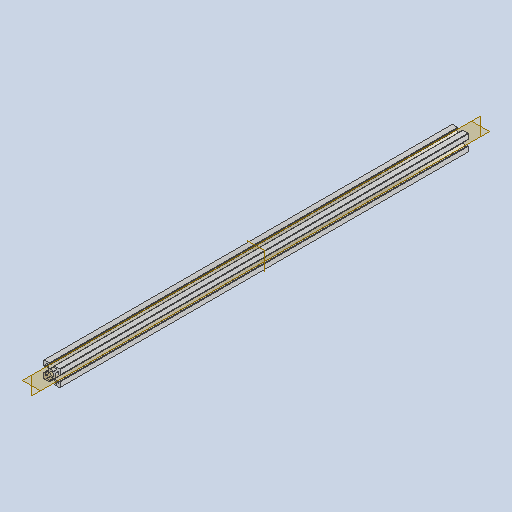
# Autodesk Inventor part: PERFIL_20X20_001
Saved by Autodesk Inventor 2026 (Build 300175000, 175)
## iProperties
Created: 2025-03-25
Part Number: PERFIL_20X20_001
Material: Alumínio 6061
Document SubType Name: Modeling
Designer: Carlos Dias
Density: 2.7 g/cm^3
Appearance: Alumínio - Polido
Description: 50x20
Author: Carlos Dias
Autodesk Inventor part; units mm, degrees
sketch "Esboço1" plane through (0, 0, 0) normal (0, 0, 1) x (1, 0, 0)
  line L0 (-10, 10) -> (10, 10) construction
  circle A0 centre (0, 0) radius 2.5
  line L1 (-4, 4) -> (4, 4) construction
  line L2 (-10, 10) -> (0, 0) construction
  line L3 (-4, 4) -> (-4, -4) construction
  line L4 (-6.5858, 8) -> (-2.5858, 4) construction
  line L5 (-6.5858, 8) -> (-2.5858, 8) construction
  line L6 (-2.5858, 8) -> (-2.5858, 10) construction
  line L7 (-2.5858, 10) -> (-3.0858, 10) construction
  line L8 (-3.0858, 10) -> (-3.0858, 9.5)
  line L9 (-3.0858, 9.5) -> (-2.5858, 9.5)
  line L10 (-2.5858, 9.5) -> (-2.5858, 10) construction
  line L11 (-8, 6.5858) -> (-4, 2.5858) construction
  line L12 (-2.5858, 8) -> (-2.5858, 9.5)
  line L13 (-3.0858, 10) -> (-10, 10)
  line L14 (-10, 10) -> (-10, 3.0858) construction
  line L15 (-10, 3.0858) -> (-8, 3.0858) construction
  line L16 (-8, 6.5858) -> (-8, 3.0858) construction
  line L17 (-10, 3.0858) -> (-9.5, 3.0858) construction
  line L18 (-9.5, 3.0858) -> (-9.5, 3.5858)
  line L19 (-9.5, 3.5858) -> (-10, 3.5858)
  line L20 (-10, 3.5858) -> (-10, 3.0858) construction
  line L21 (-8, 3.0858) -> (-9.5, 3.0858)
  arc A1 (-2.7322, 4.1464) -> (-2.3787, 4) centre (-2.3787, 4.5) ccw
  line L22 (-2.3787, 4) -> (0, 4)
  arc A2 (-5.8615, 8) -> (-6.0737, 7.4879) centre (-5.8615, 7.7) ccw
  line L23 (-6.0737, 7.4879) -> (-2.7322, 4.1464)
  line L24 (-5.8615, 8) -> (-2.5858, 8)
  arc A3 (-4, 2.3787) -> (-4.1464, 2.7322) centre (-4.5, 2.3787) ccw
  arc A4 (-7.4879, 6.0737) -> (-8, 5.8615) centre (-7.7, 5.8615) ccw
  line L25 (-8, 5.8615) -> (-8, 3.0858)
  line L26 (-7.4879, 6.0737) -> (-4.1464, 2.7322)
  arc A5 (-9.5, 10) -> (-10, 9.5) centre (-9.5, 9.5) ccw
  line L27 (-4, 2.3787) -> (-4, 0)
  line L28 (-10, 9.5) -> (-10, 3.5858)
  line L29 (-4, 0) -> (0, 0)
  line L30 (0, 4) -> (0, 0)
  point P0 (0, 10)
  point P1 (-5, 5)
  point P2 (-10, 6.5429)
  point P3 (-2.5, 0)
  point P4 (0, 2.5)
  dimension "d1" = 20
  dimension "d2" = 10
  dimension "d3" = 5
  dimension "d4" = 6
  dimension "d5" = 1
  dimension "d7" = 2
  dimension "d8" = 0.5
  dimension "d9" = 1
  dimension "d10" = 2
  dimension "d12" = 0.5
  dimension "d13" = 0.3
  dimension "d14" = 0.5
  dimension "d15" = 0.3
  dimension "d16" = 0.5
  dimension "d17" = 8
  constraints: 62 end point, 14 point on line, 10 point on circle, 10 tangent, 8 perpendicular, 7 horizontal, 6 centre point, 6 collinear, 6 parallel, 5 midpoint, 4 vertical, 3 coincident, 3 vertical alignment
  measures "d1" distance of L0.start L0.end
  measures "d2" distance from line of point (0, 0) L0
  measures "d3" diameter of A0
  measures "d4" distance between parallel lines of L1 L0
  measures "d5" distance from line of point (-5, 5) L4
  measures "d7" distance from line of L0 L4.start
  measures "d8" distance of L8.end L9.end
  measures "d9" distance between parallel lines of L2 L11
  measures "d10" distance of L14.end L15.end
  measures "d12" radius of A1
  measures "d13" radius of A2
  measures "d14" radius of A3
  measures "d15" radius of A4
  measures "d16" radius of A5
  measures "d17" distance of L1.start L1.end
extrude "Extrusão1" add sketch "Esboço1" along normal mid plane 500 contours A0 L29 L27 A3 L26 A4 L25 L21 L18 L19 L28 A5 L13 L8 L9 L12 L24 A2 L23 A1 L22 L30
mirror "Espelhar1" about plane through (0, 0, 0) normal (1, 0, 0) of "Extrusão1"
mirror "Espelhar2" about plane through (0, 0, 0) normal (0, 1, 0) of "Extrusão1", "Espelhar1"
equation "\"d2\" = 0.5 * d1"
